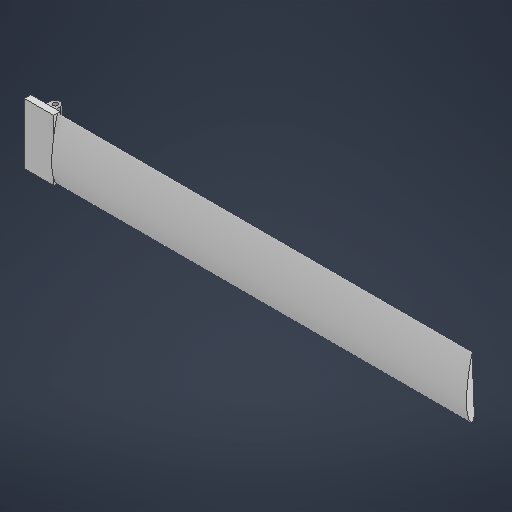
# Autodesk Inventor part: Pieza9
Saved by Autodesk Inventor 2026.1 (Build 301233000, 233)
## iProperties
Created: 2025-09-20
Part Number: Pieza9
Material: Genérico
Document SubType Name: Modeling
Designer: Usuario
Density: 1 g/cm^3
Appearance: Valor por defecto
Author: Usuario
Autodesk Inventor part; units mm, degrees
ref_plane "YZ Plane" through (0, 0, 0) normal (1, 0, 0) x (0, 1, 0)
ref_plane "XZ Plane" through (0, 0, 0) normal (0, 1, 0) x (-1, 0, 0)
ref_plane "XY Plane" through (0, 0, 0) normal (0, 0, 1) x (1, 0, 0)
sketch "Boceto1" plane through (0, 0, 0) normal (1, 0, 0) x (0, 1, 0)
  line L0 (0, 0) -> (0.3125, 0.61) construction
  line L1 (0.3125, 0.61) -> (0.625, 0.8475) construction
  line L2 (0.625, 0.8475) -> (1.25, 1.1825) construction
  line L3 (1.25, 1.1825) -> (1.875, 1.44) construction
  line L4 (1.875, 1.44) -> (2.5, 1.6475) construction
  line L5 (2.5, 1.6475) -> (3.75, 1.9725) construction
  line L6 (3.75, 1.9725) -> (5, 2.2) construction
  line L7 (5, 2.2) -> (6.25, 2.3525) construction
  line L8 (6.25, 2.3525) -> (7.5, 2.44) construction
  line L9 (7.5, 2.44) -> (10, 2.44) construction
  line L10 (10, 2.44) -> (12.5, 2.2975) construction
  line L11 (12.5, 2.2975) -> (15, 2.035) construction
  line L12 (15, 2.035) -> (17.5, 1.6725) construction
  line L13 (17.5, 1.6725) -> (20, 1.2225) construction
  line L14 (20, 1.2225) -> (22.5, 0.6775) construction
  line L15 (22.5, 0.6775) -> (23.75, 0.3675) construction
  line L16 (23.75, 0.3675) -> (25, 0.0325) construction
  line L17 (25, 0.0325) -> (25, -0.0325) construction
  line L18 (25, -0.0325) -> (23.75, -0.04) construction
  line L19 (23.75, -0.04) -> (22.5, -0.055) construction
  line L20 (22.5, -0.055) -> (20, -0.0975) construction
  line L21 (20, -0.0975) -> (17.5, -0.1625) construction
  line L22 (17.5, -0.1625) -> (15, -0.25) construction
  line L23 (15, -0.25) -> (12.5, -0.35) construction
  line L24 (12.5, -0.35) -> (10, -0.45) construction
  line L25 (10, -0.45) -> (7.5, -0.565) construction
  line L26 (7.5, -0.565) -> (6.25, -0.625) construction
  line L27 (6.25, -0.625) -> (5, -0.685) construction
  line L28 (5, -0.685) -> (3.75, -0.72) construction
  line L29 (3.75, -0.72) -> (2.5, -0.72) construction
  line L30 (2.5, -0.72) -> (1.875, -0.685) construction
  line L31 (1.875, -0.685) -> (1.25, -0.6225) construction
  line L32 (1.25, -0.6225) -> (0.625, -0.4875) construction
  line L33 (0.625, -0.4875) -> (0.3125, -0.3575) construction
  line L34 (0.3125, -0.3575) -> (0, 0) construction
  spline S0 degree 4 poles (0, 0) (0.3125, 0.61) (0.625, 0.8475) (1.25, 1.1825) (1.875, 1.44) (2.5, 1.6475) (3.75, 1.9725) (5, 2.2) (6.25, 2.3525) (7.5, 2.44) (10, 2.44) (12.5, 2.2975) (15, 2.035) (17.5, 1.6725) (20, 1.2225) (22.5, 0.6775) (23.75, 0.3675) (25, 0.0325) (25, -0.0325) (23.75, -0.04) (22.5, -0.055) (20, -0.0975) (17.5, -0.1625) (15, -0.25) (12.5, -0.35) (10, -0.45) (7.5, -0.565) (6.25, -0.625) (5, -0.685) (3.75, -0.72) (2.5, -0.72) (1.875, -0.685) (1.25, -0.6225) (0.625, -0.4875) (0.3125, -0.3575) (0, 0) knots 1 1 1 1 1 2 3 4 5 6 7 8 9 10 11 12 13 14 15 16 17 18 19 20 21 22 23 24 25 26 27 28 29 30 31 32 33 33 33 33 33
  constraints: 34 coincident, 2 horizontal, 1 vertical, 2 other
extrude "Extrusión1" add sketch "Boceto1" along normal blind 170
sketch "Boceto2" plane through (0, 0, 0) normal (-1, 0, 0) x (0, 0, 1)
  line L0 (0.2928, 24.8849) -> (-1.0423, 24.8849)
  line L1 (-1.0423, 24.8849) -> (-1.0423, 0)
  line L2 (-1.0423, 0) -> (0.2928, 0)
  line L3 (0.2928, 0) -> (0.2928, 24.8849) construction
  line L4 (1.6279, 24.8849) -> (1.6279, 0)
  line L5 (1.6279, 0) -> (0.2928, 0)
  line L6 (0.2928, 24.8849) -> (1.6279, 24.8849)
  point P0 (0, 0)
  constraints: 14 end point, 2 parallel, 2 symmetric about line, 1 horizontal, 1 perpendicular
extrude "Extrusión2" add sketch "Boceto2" along normal blind 12
sketch "Boceto3" plane through (0, 0, -1.0423) normal (0, 0, -1) x (-1, 0, 0)
  line L0 (12.002, 24.8986) -> (0, 0) construction
  line L1 (0, 24.8986) -> (12.002, 0) construction
  line L2 (6.001, 12.4493) -> (6.001, 7.3493) construction
  line L3 (6.001, 7.3493) -> (8.001, 7.3493)
  line L4 (8.001, 7.3493) -> (8.001, 2.3493)
  line L5 (8.001, 2.3493) -> (6.001, 2.3493)
  line L6 (6.001, 2.3493) -> (6.001, 7.3493) construction
  line L7 (6.001, 7.3493) -> (4.001, 7.3493)
  line L8 (4.001, 7.3493) -> (4.001, 2.3493)
  line L9 (4.001, 2.3493) -> (6.001, 2.3493)
  line L10 (8.4032, 12.4493) -> (2.616, 12.4493) construction
  line L11 (12.002, 0) -> (0, 24.8986) construction
  line L12 (0, 0) -> (12.002, 24.8986) construction
  line L13 (6.001, 12.4493) -> (6.001, 17.5493) construction
  line L14 (6.001, 17.5493) -> (8.001, 17.5493)
  line L15 (8.001, 17.5493) -> (8.001, 22.5493)
  line L16 (8.001, 22.5493) -> (6.001, 22.5493)
  line L17 (6.001, 22.5493) -> (6.001, 17.5493) construction
  line L18 (6.001, 17.5493) -> (4.001, 17.5493)
  line L19 (4.001, 17.5493) -> (4.001, 22.5493)
  line L20 (4.001, 22.5493) -> (6.001, 22.5493)
  dimension "d4" = 5.1
  dimension "d5" = 2
  dimension "d6" = 5
  constraints: 42 end point, 12 symmetric about line, 2 horizontal, 2 parallel, 1 perpendicular, 1 vertical
  measures "d4" distance of L2.start L2.end
  measures "d5" distance of L4.end L5.end
  measures "d6" distance of L3.end L4.end
extrude "Extrusión3" add sketch "Boceto3" along normal blind 6
sketch "Boceto4" plane through (-8.001, 22.5493, -1.0423) normal (0, 1, 0) x (1, 0, 0)
  line L0 (4, 0) -> (4, 6) construction
  line L1 (0, 6) -> (4, 6) construction
  line L2 (4, 0) -> (0, 0) construction
  line L3 (0, 0) -> (0, 6) construction
  line L4 (0, 6) -> (4, 6) construction
  line L5 (4, 6) -> (4, 0) construction
  circle A0 centre (2, 4) radius 1
  line L6 (0, 6) -> (4, 6)
  line L7 (4, 6) -> (4, 2)
  line L8 (4, 2) -> (0, 2) construction
  line L9 (0, 2) -> (0, 6) construction
  point P0 (8.001, -1.0423)
  dimension "d9" = 2
  dimension "d13" = 4
  dimension "d14" = 4
  constraints: 16 end point, 4 parallel, 2 horizontal, 2 perpendicular, 1 centre point
  measures "d9" diameter of A0
  measures "d13" distance of L7.end L8.end
  measures "d14" distance of L6.end L7.end
extrude "Extrusión4" cut sketch "Boceto4" against normal through all
fillet "Empalme1" radius 2 4 edges at (-8.001, 20.0493, -7.0423) (-4.001, 20.0493, -7.0423) (-8.001, 4.8493, -7.0423) (-4.001, 4.8493, -7.0423)
